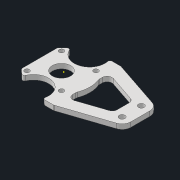
# Autodesk Inventor part: pistonplatefront
Saved by Autodesk Inventor 2022 (Build 260153000, 153)
## iProperties
Created: 2022-09-21
Part Number: pistonplatefront
Material: Generic
Document SubType Name: Modeling
Designer: Kieran Jarvis
Density: 1 g/cm^3
Appearance: Default
Author: Kieran Jarvis
Autodesk Inventor part; units mm, degrees
ref_plane "YZ Plane" through (0, 0, 0) normal (1, 0, 0) x (0, 1, 0)
ref_plane "XZ Plane" through (0, 0, 0) normal (0, 1, 0) x (-1, 0, 0)
ref_plane "XY Plane" through (0, 0, 0) normal (0, 0, 1) x (1, 0, 0)
sketch "Sketch1" plane through (0, 0, 0) normal (0, 1, 0) x (-1, 0, 0)
  circle A0 centre (2.2, 0) radius 9.525 projected
  circle A1 centre (-15.7605, -17.9605) radius 2.0193 construction
  circle A2 centre (20.1605, -17.9605) radius 2.0193 construction
  circle A3 centre (20.1605, 17.9605) radius 2.0193 construction
  circle A4 centre (-15.7605, 17.9605) radius 2.0193 construction
  circle A5 centre (2.2, -29.26) radius 15.5575 construction
  circle A6 centre (2.2, 29.26) radius 15.5575 construction
  circle A7 centre (-71, 10) radius 3 construction
  circle A8 centre (-71, -10) radius 3 construction
  line L0 (-93.1199, -15.5417) -> (-49.1294, -16.4557) construction
  line L1 (-49.1294, -16.4557) -> (-48.8801, -4.4583) construction
  line L2 (-92.8706, -3.5443) -> (-48.8801, -4.4583) construction
  line L3 (-93.1199, -15.5417) -> (-92.8706, -3.5443) construction
  line L4 (-25, 210) -> (-25, -210) construction
  line L5 (25, 210) -> (25, -210) construction
  arc A9 (17.6544, -25.1175) -> (-13.2881, -25.2451) centre (2.2, -29.26) ccw
  circle A10 centre (-71, -10) radius 9 construction
  circle A11 centre (-71, 10) radius 9 construction
  line L6 (23, -35) -> (-24.672, -35) construction
  line L7 (-24.672, 35) -> (23, 35) construction
  line L8 (25, -18.7054) -> (25, 18.7057)
  arc A12 (17.6544, -25.1175) -> (25, -18.7054) centre (2.2, 0) ccw
  arc A13 (-13.2544, -25.1175) -> (-12.7349, -35) centre (2.2, -29.26) ccw
  arc A14 (-12.7349, 35) -> (17.6545, 25.1177) centre (2.2, 29.26) ccw
  arc A15 (25, 18.7057) -> (17.6545, 25.1177) centre (2.2, 0) ccw
  line L9 (-12.7349, -35) -> (-24.672, -35)
  line L10 (-12.7349, 35) -> (-24.672, 35)
  line L11 (-24.672, -35) -> (-73.8571, -18.5345)
  line L12 (-24.672, 35) -> (-73.8571, 18.5345)
  line L13 (-80, -10) -> (-80, 10)
  arc A16 (-80, -10) -> (-73.8571, -18.5345) centre (-71, -10) ccw
  arc A17 (-73.8571, 18.5345) -> (-80, 10) centre (-71, 10) ccw
  line L14 (-58.5968, -11.0143) -> (-31.5968, -20.1136) projected
  arc A18 (-62, -6.2761) -> (-58.5968, -11.0143) centre (-57, -6.2761) ccw projected
  line L15 (-62, 6.2761) -> (-62, -6.2761) projected
  arc A19 (-58.5968, 11.0143) -> (-62, 6.2761) centre (-57, 6.2761) ccw projected
  line L16 (-31.5968, 20.1136) -> (-58.5968, 11.0143) projected
  arc A20 (-25, 15.3755) -> (-31.5968, 20.1136) centre (-30, 15.3755) ccw projected
  arc A21 (-31.5968, -20.1136) -> (-25, -15.3755) centre (-30, -15.3755) ccw projected
  arc A22 (-25, 11.397) -> (-25, -11.397) centre (2.2, 0) ccw
  line L17 (-25, -15.3755) -> (-25, -11.397)
  line L18 (-25, 15.3755) -> (-25, 11.397)
  arc A23 (-18.6534, -20.8534) -> (23.0534, 20.8534) centre (2.2, 0) ccw projected
  spline S0 degree 3 poles (23.0534, 20.8534) (21.798, 22.1089) (20.4403, 23.2417) (18.9803, 24.2518) (18.9572, 24.2679) (18.9354, 24.2829) (18.9107, 24.2998) (17.3595, 25.3666) (15.7211, 26.2765) (13.9955, 27.0296) (13.9681, 27.0415) (13.9418, 27.0529) (13.9132, 27.0653) (12.1415, 27.8321) (10.3123, 28.4192) (8.4258, 28.8266) (8.3649, 28.8397) (8.3053, 28.8524) (8.243, 28.8654) (6.2506, 29.2826) (4.2356, 29.4912) (2.2, 29.4912) (0.228, 29.4912) (-1.724, 29.2955) (-3.6561, 28.9039) (-3.7184, 28.8913) (-3.7821, 28.8782) (-3.843, 28.8654) (-5.7631, 28.4635) (-7.6246, 27.8758) (-9.4274, 27.1023) (-9.456, 27.09) (-9.4858, 27.0772) (-9.5132, 27.0653) (-11.241, 26.3176) (-12.8822, 25.4127) (-14.4368, 24.3505) (-14.4614, 24.3337) (-14.4875, 24.3158) (-14.5107, 24.2998) (-15.9968, 23.278) (-17.3782, 22.1287) (-18.6534, 20.8534) (-19.9088, 19.5981) (-21.0416, 18.2404) (-22.0518, 16.7803) (-22.0679, 16.7572) (-22.0829, 16.7354) (-22.0998, 16.7107) (-23.1666, 15.1595) (-24.0765, 13.5211) (-24.8296, 11.7955) (-24.8415, 11.7681) (-24.8529, 11.7418) (-24.8653, 11.7132) (-25.6321, 9.9415) (-26.2192, 8.1123) (-26.6266, 6.2258) (-26.6397, 6.1649) (-26.6524, 6.1053) (-26.6654, 6.043) (-27.0826, 4.0506) (-27.2912, 2.0356) (-27.2912, 0) (-27.2912, -1.972) (-27.0955, -3.924) (-26.7039, -5.8561) (-26.6913, -5.9184) (-26.6782, -5.9821) (-26.6654, -6.043) (-26.2635, -7.9631) (-25.6758, -9.8246) (-24.9023, -11.6274) (-24.89, -11.656) (-24.8772, -11.6858) (-24.8653, -11.7132) (-24.1176, -13.441) (-23.2127, -15.0822) (-22.1505, -16.6368) (-22.1337, -16.6614) (-22.1158, -16.6875) (-22.0998, -16.7107) (-21.0779, -18.1969) (-19.929, -19.5778) (-18.6534, -20.8534) knots 0 0 0 0 0.061523 0.061523 0.061523 0.0625 0.0625 0.0625 0.124023 0.124023 0.124023 0.125 0.125 0.125 0.185547 0.185547 0.185547 0.1875 0.1875 0.1875 0.25 0.25 0.25 0.310547 0.310547 0.310547 0.3125 0.3125 0.3125 0.374023 0.374023 0.374023 0.375 0.375 0.375 0.436523 0.436523 0.436523 0.4375 0.4375 0.4375 0.5 0.5 0.5 0.561523 0.561523 0.561523 0.5625 0.5625 0.5625 0.624023 0.624023 0.624023 0.625 0.625 0.625 0.685547 0.685547 0.685547 0.6875 0.6875 0.6875 0.75 0.75 0.75 0.810547 0.810547 0.810547 0.8125 0.8125 0.8125 0.874023 0.874023 0.874023 0.875 0.875 0.875 0.936523 0.936523 0.936523 0.9375 0.9375 0.9375 1 1 1 1 projected
  point P0 (0, 0)
  point P1 (-13.2881, -25.2451)
  dimension "d4" = 16
  dimension "d5" = 18
  dimension "d6" = 18
  dimension "d7" = 16
  constraints: 22 point on circle, 16 end point, 10 centre point, 10 coincident, 5 tangent, 2 collinear, 2 point on line, 1 parallel, 1 vertical, 10 other
  measures "d4" radius of A9
  measures "d5" diameter of A10
  measures "d6" diameter of A11
  measures "d7" radius of A14
extrude "Extrusion1" add sketch "Sketch1" against normal blind 5 contours A9 A23 S0 A22 A14 A15 L8 A12 | A9 A13 L9 L11 A16 L13 A17 L12 L10 A14 S0 L18 A20 L16 A19 L15 A18 L14 A21 L17 A23
fillet "Fillet1" radius 5 2 edges at (25, -2.5, 11.397) (25, -2.5, -11.397)
fillet "Fillet2" radius 2 8 edges at (12.7349, -2.5, 35) (-17.6545, -2.5, 25.1177) (-17.6544, -2.5, -25.1175) (12.7349, -2.5, -35) (24.672, -2.5, -35) (24.672, -2.5, 35) (-25, -2.5, -18.7054) (-25, -2.5, 18.7057)
sketch "Sketch2" plane through (0, 0, 0) normal (0, 1, 0) x (1, 0, 0)
  circle A0 centre (71, 10) radius 3 projected
  circle A1 centre (71, -10) radius 3 projected
  point P0 (0, 0)
hole "Hole1" at (71, 0, -10) at (71, 0, 10) direction (0, -1, 0) diameter 6 end through all
sketch "Sketch3" plane through (0, 0, 0) normal (0, 1, 0) x (1, 0, 0)
  point P0 (0, 0)
sketch "Sketch4" plane through (0, 0, 0) normal (0, 1, 0) x (1, 0, 0)
  circle A0 centre (-20.1605, -17.9605) radius 3 projected
  circle A1 centre (15.7605, 17.9605) radius 3 projected
  circle A2 centre (15.7605, -17.9605) radius 3 projected
  circle A3 centre (-20.1605, 17.9605) radius 3 projected
  circle A4 centre (-4, -61.01) radius 14.2875 projected
  circle A5 centre (-2.2, 29.26) radius 14.2875 projected
  circle A6 centre (-2.2, -29.26) radius 14.2875 projected
  circle A7 centre (-4, 61.01) radius 14.2875 projected
  circle A8 centre (-2.2, 0) radius 9.5 projected
  line L0 (-25, -210) -> (25, -210) projected
  line L1 (25, -210) -> (25, 210) projected
  line L2 (-25, 210) -> (25, 210) projected
  line L3 (-25, -210) -> (-25, 210) projected
  point P0 (0, 0)
  constraints: 4 coincident
hole "Hole2" at (15.7605, 0, -17.9605) at (15.7605, 0, 17.9605) at (-20.1605, 0, 17.9605) at (-20.1605, 0, -17.9605) direction (0, -1, 0) diameter 5 depth 8 tip angle 118
body "Solid1"
